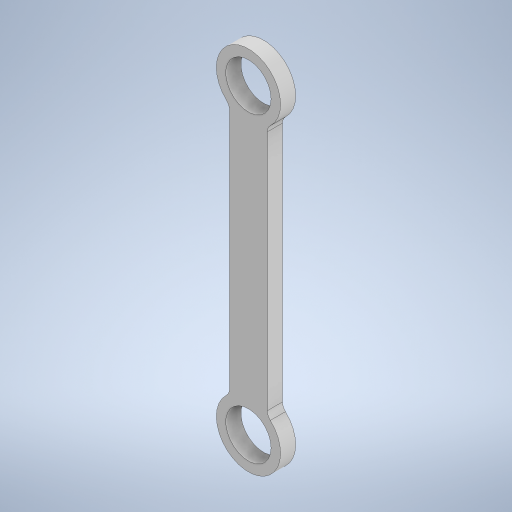
# Autodesk Inventor part: RP_Thigh-Link
Saved by Autodesk Inventor 2024.3 (Build 283343000, 343)
## iProperties
Created: 2024-10-20
Part Number: RP_Thigh-Link
Material: アルミニウム7075
Document SubType Name: Modeling
Designer: 佐藤智貴
Density: 2.8 g/cm^3
Appearance: 一般
Mass: 77.681 g
Surface Area: 116.244 cm^2
Volume: 27.7432 cm^3
Author: 佐藤智貴
Autodesk Inventor part; units mm, degrees
ref_plane "YZ Plane" through (0, 0, 0) normal (1, 0, 0) x (0, 1, 0)
ref_plane "XZ Plane" through (0, 0, 0) normal (0, 1, 0) x (-1, 0, 0)
ref_plane "XY Plane" through (0, 0, 0) normal (0, 0, 1) x (1, 0, 0)
sketch "スケッチ1" plane through (0, 0, 0) normal (0, 0, 1) x (1, 0, 0)
  circle A0 centre (0, 0) radius 17
  circle A1 centre (0, 0) radius 12
  circle A2 centre (0, -160) radius 12
  line L0 (-12, 0) -> (10.75, 0)
  line L1 (12, -160) -> (11, -160)
  circle A3 centre (0, -160) radius 17
  line L2 (-10, 24.6876) -> (10, 24.6876)
  line L3 (10, 24.6876) -> (10, -208.9864)
  line L4 (10, -208.9864) -> (-10, -208.9864)
  line L5 (-10, -208.9864) -> (-10, 24.6876)
  point P0 (-8, 8.9443)
  point P1 (12, 0)
  point P2 (0, -167.6676)
  point P3 (9.375, -145.8187)
  point P4 (-10.625, -146.7294)
  point P5 (-10.625, -13.2706)
  point P6 (9.375, -14.1813)
  point P7 (-0.625, 0)
  point P8 (-10, -13.7477)
  point P9 (-10, -146.2523)
  point P10 (10, -146.2523)
  point P11 (10, -13.7477)
  point P12 (10, -173.7477)
  point P13 (-10, -173.7477)
  point P14 (-10, 13.7477)
  point P15 (10, 13.7477)
  point P16 (-10, 6.6332)
  point P17 (-10, 0)
  point P18 (10, 0)
  point P19 (10, 6.6332)
  point P20 (-10, -6.6332)
  point P21 (10, -6.6332)
  point P22 (-10, -153.3668)
  point P23 (-10, -166.6332)
  point P24 (10, -166.6332)
  point P25 (10, -153.3668)
  dimension "d17" = 24
  dimension "d0" = 34
  dimension "d1" = 24
  dimension "d22" = 160
  dimension "d24" = 0
  dimension "d27" = 34
  dimension "d31" = 10
  dimension "d32" = 20
  constraints: 12 end point, 7 point on circle, 3 centre point, 3 parallel, 2 horizontal, 1 coincident, 1 midpoint, 1 perpendicular, 3 other
  measures "d0" diameter of A0
  measures "d1" diameter of A1
  measures "d22" distance of A3.centre A0.centre
  measures "d24" horizontal distance of point (0, -167.668) A3.centre
  measures "d27" diameter of A3
  measures "d31" distance from line of A0.centre L5
  measures "d32" distance of L2.start L2.end
extrude "押し出し1" add sketch "スケッチ1" along normal blind 8 contours A0 L3 A1 | L3 A1 L5 A0 | L3 A3 L5 A0 | A0 L5 A1 L3 | L5 A1 A0 | L3 A2 L5 A3 | A3 L3 A2 | L5 A2 A3 | L5 A2 L3 A3
fillet "フィレット2" radius 5 4 edges at (-10, -146.2523, 4) (10, -146.2523, 4) (10, -13.7477, 4) (-10, -13.7477, 4)
equation "\"d17\" = d1"
equation "\"d31\" = 0.5 * d32"
equation "\"d23\" = 0.5 * d3"
equation "\"d3\" = 10"
